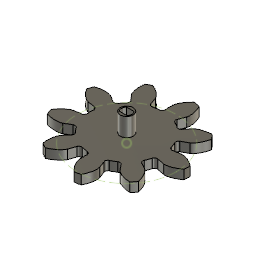
Master Gear (Autodesk Fusion 360 design; units mm, degrees)
description: Spur Gear; Module: 6.000000; Num Teeth: 9; Pressure Angle: 20.000000; Backlash: 0.00 mm
Autodesk Fusion 360 part; units mm, degrees
(part 1 of 2)
sketch "Sketch1" plane through (0, 0, 0) normal (0, 0, 1) x (1, 0, 0) in component "Spur Gear (9 teeth)"
  circle A0 centre (0, 0) radius 19.7492
extrude "Extrude1" add sketch "Sketch1" along normal blind 5 in component "Spur Gear (9 teeth)"
sketch "Sketch2" plane through (0, 0, 0) normal (0, 0, 1) x (1, 0, 0) in component "Spur Gear (9 teeth)"
  spline S0 degree 5 poles (24.9178, -4.7777) (24.9406, -4.782) (24.9862, -4.7899) (25.0549, -4.7992) (25.1471, -4.8069) (25.263, -4.8101) (25.3794, -4.8088) (25.4962, -4.8047) (25.6131, -4.7991) (25.7301, -4.7925) (25.8472, -4.7846) (25.9644, -4.7752) (26.0817, -4.7637) (26.1992, -4.7499) (26.3168, -4.7338) (26.4345, -4.7156) (26.5523, -4.6956) (26.67, -4.6741) (26.7878, -4.6513) (26.9056, -4.6272) (27.0233, -4.6018) (27.1411, -4.5751) (27.2588, -4.5468) (27.3765, -4.5171) (27.4941, -4.486) (27.6117, -4.4534) (27.7292, -4.4196) (27.8467, -4.3845) (27.9641, -4.3482) (28.0813, -4.3107) (28.1985, -4.272) (28.3156, -4.2321) (28.4326, -4.191) (28.5495, -4.1487) (28.6662, -4.1053) (28.7828, -4.0606) (28.8993, -4.0149) (29.0157, -3.968) (29.1319, -3.9201) (29.2479, -3.8711) (29.3638, -3.821) (29.4795, -3.7698) (29.595, -3.7175) (29.7104, -3.6643) (29.8256, -3.6099) (29.9406, -3.5546) (30.0554, -3.4982) (30.17, -3.4408) (30.2844, -3.3824) (30.3986, -3.323) (30.5125, -3.2626) (30.6263, -3.2013) (30.7398, -3.139) (30.8531, -3.0757) (30.9662, -3.0114) (31.079, -2.9462) (31.1916, -2.8801) (31.3039, -2.8131) (31.416, -2.7451) (31.5279, -2.6762) (31.6394, -2.6063) (31.7507, -2.5356) (31.8618, -2.464) (31.9725, -2.3914) (32.083, -2.318) (32.1932, -2.2437) (32.3031, -2.1685) (32.4127, -2.0925) (32.522, -2.0156) (32.6311, -1.9378) (32.7398, -1.8592) (32.8265, -1.7956) (32.8914, -1.7475) (32.9346, -1.7153) (32.9562, -1.6991) knots 0 0 0 0 0 0 0.01428571 0.02857143 0.04285714 0.05714286 0.07142857 0.08571429 0.1 0.11428571 0.12857143 0.14285714 0.15714286 0.17142857 0.18571429 0.2 0.21428571 0.22857143 0.24285714 0.25714286 0.27142857 0.28571429 0.3 0.31428571 0.32857143 0.34285714 0.35714286 0.37142857 0.38571429 0.4 0.41428571 0.42857143 0.44285714 0.45714286 0.47142857 0.48571429 0.5 0.51428571 0.52857143 0.54285714 0.55714286 0.57142857 0.58571429 0.6 0.61428571 0.62857143 0.64285714 0.65714286 0.67142857 0.68571429 0.7 0.71428571 0.72857143 0.74285714 0.75714286 0.77142857 0.78571429 0.8 0.81428571 0.82857143 0.84285714 0.85714286 0.87142857 0.88571429 0.9 0.91428571 0.92857143 0.94285714 0.95714286 0.97142857 0.98571429 1 1 1 1 1 1
  spline S1 degree 5 poles (24.9178, 4.7777) (24.9406, 4.782) (24.9862, 4.7899) (25.0549, 4.7992) (25.1471, 4.8069) (25.263, 4.8101) (25.3794, 4.8088) (25.4962, 4.8047) (25.6131, 4.7991) (25.7301, 4.7925) (25.8472, 4.7846) (25.9644, 4.7752) (26.0817, 4.7637) (26.1992, 4.7499) (26.3168, 4.7338) (26.4345, 4.7156) (26.5523, 4.6956) (26.67, 4.6741) (26.7878, 4.6513) (26.9056, 4.6272) (27.0233, 4.6018) (27.1411, 4.5751) (27.2588, 4.5468) (27.3765, 4.5171) (27.4941, 4.486) (27.6117, 4.4534) (27.7292, 4.4196) (27.8467, 4.3845) (27.9641, 4.3482) (28.0813, 4.3107) (28.1985, 4.272) (28.3156, 4.2321) (28.4326, 4.191) (28.5495, 4.1487) (28.6662, 4.1053) (28.7828, 4.0606) (28.8993, 4.0149) (29.0157, 3.968) (29.1319, 3.9201) (29.2479, 3.8711) (29.3638, 3.821) (29.4795, 3.7698) (29.595, 3.7175) (29.7104, 3.6643) (29.8256, 3.6099) (29.9406, 3.5546) (30.0554, 3.4982) (30.17, 3.4408) (30.2844, 3.3824) (30.3986, 3.323) (30.5125, 3.2626) (30.6263, 3.2013) (30.7398, 3.139) (30.8531, 3.0757) (30.9662, 3.0114) (31.079, 2.9462) (31.1916, 2.8801) (31.3039, 2.8131) (31.416, 2.7451) (31.5279, 2.6762) (31.6394, 2.6063) (31.7507, 2.5356) (31.8618, 2.464) (31.9725, 2.3914) (32.083, 2.318) (32.1932, 2.2437) (32.3031, 2.1685) (32.4127, 2.0925) (32.522, 2.0156) (32.6311, 1.9378) (32.7398, 1.8592) (32.8265, 1.7956) (32.8914, 1.7475) (32.9346, 1.7153) (32.9562, 1.6991) knots 0 0 0 0 0 0 0.01428571 0.02857143 0.04285714 0.05714286 0.07142857 0.08571429 0.1 0.11428571 0.12857143 0.14285714 0.15714286 0.17142857 0.18571429 0.2 0.21428571 0.22857143 0.24285714 0.25714286 0.27142857 0.28571429 0.3 0.31428571 0.32857143 0.34285714 0.35714286 0.37142857 0.38571429 0.4 0.41428571 0.42857143 0.44285714 0.45714286 0.47142857 0.48571429 0.5 0.51428571 0.52857143 0.54285714 0.55714286 0.57142857 0.58571429 0.6 0.61428571 0.62857143 0.64285714 0.65714286 0.67142857 0.68571429 0.7 0.71428571 0.72857143 0.74285714 0.75714286 0.77142857 0.78571429 0.8 0.81428571 0.82857143 0.84285714 0.85714286 0.87142857 0.88571429 0.9 0.91428571 0.92857143 0.94285714 0.95714286 0.97142857 0.98571429 1 1 1 1 1 1
  arc A0 (32.9562, -1.6991) -> (32.9562, 1.6991) centre (0, 0) ccw
  line L0 (19.3861, -3.7189) -> (24.9178, -4.7777)
  line L1 (19.3861, 3.7189) -> (24.9178, 4.7777)
  line L2 (19.3861, -3.7189) -> (19.3861, 3.7189)
  point P0 (25.4672, -4.8054)
  point P1 (26.0282, -4.7687)
  point P2 (26.5965, -4.6873)
  point P3 (27.1699, -4.5679)
  point P4 (27.7472, -4.414)
  point P5 (28.3272, -4.2278)
  point P6 (28.909, -4.0108)
  point P7 (29.4915, -3.7641)
  point P8 (30.0739, -3.4887)
  point P9 (30.6555, -3.1851)
  point P10 (31.2353, -2.8539)
  point P11 (31.8125, -2.4956)
  point P12 (32.3864, -2.1106)
  point P13 (25.4672, 4.8054)
  point P14 (26.0282, 4.7687)
  point P15 (26.5965, 4.6873)
  point P16 (27.1699, 4.5679)
  point P17 (27.7472, 4.414)
  point P18 (28.3272, 4.2278)
  point P19 (28.909, 4.0108)
  point P20 (29.4915, 3.7641)
  point P21 (30.0739, 3.4887)
  point P22 (30.6555, 3.1851)
  point P23 (31.2353, 2.8539)
  point P24 (31.8125, 2.4956)
  point P25 (32.3864, 2.1106)
extrude "Extrude2" add sketch "Sketch2" along normal blind 5 in component "Spur Gear (9 teeth)"
fillet "Fillet1" radius 1.5875 2 edges at (19.3955, -3.7207, 2.5) (19.3955, 3.7207, 2.5) in component "Spur Gear (9 teeth)"
pattern_circular "C-Pattern1" count 9 over 360 about axis through (0, 0, 0) along (0, 0, 1) of "Extrude2", "Fillet1" in component "Spur Gear (9 teeth)"
sketch "Sketch3" plane through (0, 0, 0) normal (0, 0, 1) x (1, 0, 0) in component "Spur Gear (9 teeth)"
  circle A0 centre (0, 0) radius 27 construction
sketch "Sketch1 (2)" plane through (0, 0, 5) normal (0, 0, 1) x (-1, 0, 0)
  arc A0 (-17.9169, 8.3075) -> (-19.0651, 5.1529) centre (0, 0) ccw
  arc A1 (-20.896, 4.0079) -> (-19.0651, 5.1529) centre (-20.5976, 5.5671) ccw
  line L0 (-20.896, 4.0079) -> (-24.9178, 4.7777)
  spline S0 degree 5 poles (-24.9178, 4.7777) (-24.9406, 4.782) (-24.9862, 4.7899) (-25.0549, 4.7992) (-25.1471, 4.8069) (-25.263, 4.8101) (-25.3794, 4.8088) (-25.4962, 4.8047) (-25.6131, 4.7991) (-25.7301, 4.7925) (-25.8472, 4.7846) (-25.9644, 4.7752) (-26.0817, 4.7637) (-26.1992, 4.7499) (-26.3168, 4.7338) (-26.4345, 4.7156) (-26.5523, 4.6956) (-26.67, 4.6741) (-26.7878, 4.6513) (-26.9056, 4.6272) (-27.0233, 4.6018) (-27.1411, 4.5751) (-27.2588, 4.5468) (-27.3765, 4.5171) (-27.4941, 4.486) (-27.6117, 4.4534) (-27.7292, 4.4196) (-27.8467, 4.3845) (-27.9641, 4.3482) (-28.0813, 4.3107) (-28.1985, 4.272) (-28.3156, 4.2321) (-28.4326, 4.191) (-28.5495, 4.1487) (-28.6662, 4.1053) (-28.7828, 4.0606) (-28.8993, 4.0149) (-29.0157, 3.968) (-29.1319, 3.9201) (-29.2479, 3.8711) (-29.3638, 3.821) (-29.4795, 3.7698) (-29.595, 3.7175) (-29.7104, 3.6643) (-29.8256, 3.6099) (-29.9406, 3.5546) (-30.0554, 3.4982) (-30.17, 3.4408) (-30.2844, 3.3824) (-30.3986, 3.323) (-30.5125, 3.2626) (-30.6263, 3.2013) (-30.7398, 3.139) (-30.8531, 3.0757) (-30.9662, 3.0114) (-31.079, 2.9462) (-31.1916, 2.8801) (-31.3039, 2.8131) (-31.416, 2.7451) (-31.5279, 2.6762) (-31.6394, 2.6063) (-31.7507, 2.5356) (-31.8618, 2.464) (-31.9725, 2.3914) (-32.083, 2.318) (-32.1932, 2.2437) (-32.3031, 2.1685) (-32.4127, 2.0925) (-32.522, 2.0156) (-32.6311, 1.9378) (-32.7398, 1.8592) (-32.8265, 1.7956) (-32.8914, 1.7475) (-32.9346, 1.7153) (-32.9562, 1.6991) knots 0 0 0 0 0 0 0.01428571 0.02857143 0.04285714 0.05714286 0.07142857 0.08571429 0.1 0.11428571 0.12857143 0.14285714 0.15714286 0.17142857 0.18571429 0.2 0.21428571 0.22857143 0.24285714 0.25714286 0.27142857 0.28571429 0.3 0.31428571 0.32857143 0.34285714 0.35714286 0.37142857 0.38571429 0.4 0.41428571 0.42857143 0.44285714 0.45714286 0.47142857 0.48571429 0.5 0.51428571 0.52857143 0.54285714 0.55714286 0.57142857 0.58571429 0.6 0.61428571 0.62857143 0.64285714 0.65714286 0.67142857 0.68571429 0.7 0.71428571 0.72857143 0.74285714 0.75714286 0.77142857 0.78571429 0.8 0.81428571 0.82857143 0.84285714 0.85714286 0.87142857 0.88571429 0.9 0.91428571 0.92857143 0.94285714 0.95714286 0.97142857 0.98571429 1 1 1 1 1 1
  arc A2 (-32.9562, 1.6991) -> (-32.9562, -1.6991) centre (0, 0) ccw
  spline S1 degree 5 poles (-32.9562, -1.6991) (-32.9346, -1.7153) (-32.8914, -1.7475) (-32.8265, -1.7956) (-32.7398, -1.8592) (-32.6311, -1.9378) (-32.522, -2.0156) (-32.4127, -2.0925) (-32.3031, -2.1685) (-32.1932, -2.2437) (-32.083, -2.318) (-31.9725, -2.3914) (-31.8618, -2.464) (-31.7507, -2.5356) (-31.6394, -2.6063) (-31.5279, -2.6762) (-31.416, -2.7451) (-31.3039, -2.8131) (-31.1916, -2.8801) (-31.079, -2.9462) (-30.9662, -3.0114) (-30.8531, -3.0757) (-30.7398, -3.139) (-30.6263, -3.2013) (-30.5125, -3.2626) (-30.3986, -3.323) (-30.2844, -3.3824) (-30.17, -3.4408) (-30.0554, -3.4982) (-29.9406, -3.5546) (-29.8256, -3.6099) (-29.7104, -3.6643) (-29.595, -3.7175) (-29.4795, -3.7698) (-29.3638, -3.821) (-29.2479, -3.8711) (-29.1319, -3.9201) (-29.0157, -3.968) (-28.8993, -4.0149) (-28.7828, -4.0606) (-28.6662, -4.1053) (-28.5495, -4.1487) (-28.4326, -4.191) (-28.3156, -4.2321) (-28.1985, -4.272) (-28.0813, -4.3107) (-27.9641, -4.3482) (-27.8467, -4.3845) (-27.7292, -4.4196) (-27.6117, -4.4534) (-27.4941, -4.486) (-27.3765, -4.5171) (-27.2588, -4.5468) (-27.1411, -4.5751) (-27.0233, -4.6018) (-26.9056, -4.6272) (-26.7878, -4.6513) (-26.67, -4.6741) (-26.5523, -4.6956) (-26.4345, -4.7156) (-26.3168, -4.7338) (-26.1992, -4.7499) (-26.0817, -4.7637) (-25.9644, -4.7752) (-25.8472, -4.7846) (-25.7301, -4.7925) (-25.6131, -4.7991) (-25.4962, -4.8047) (-25.3794, -4.8088) (-25.263, -4.8101) (-25.1471, -4.8069) (-25.0549, -4.7992) (-24.9862, -4.7899) (-24.9406, -4.782) (-24.9178, -4.7777) knots -1 -1 -1 -1 -1 -1 -0.98571429 -0.97142857 -0.95714286 -0.94285714 -0.92857143 -0.91428571 -0.9 -0.88571429 -0.87142857 -0.85714286 -0.84285714 -0.82857143 -0.81428571 -0.8 -0.78571429 -0.77142857 -0.75714286 -0.74285714 -0.72857143 -0.71428571 -0.7 -0.68571429 -0.67142857 -0.65714286 -0.64285714 -0.62857143 -0.61428571 -0.6 -0.58571429 -0.57142857 -0.55714286 -0.54285714 -0.52857143 -0.51428571 -0.5 -0.48571429 -0.47142857 -0.45714286 -0.44285714 -0.42857143 -0.41428571 -0.4 -0.38571429 -0.37142857 -0.35714286 -0.34285714 -0.32857143 -0.31428571 -0.3 -0.28571429 -0.27142857 -0.25714286 -0.24285714 -0.22857143 -0.21428571 -0.2 -0.18571429 -0.17142857 -0.15714286 -0.14285714 -0.12857143 -0.11428571 -0.1 -0.08571429 -0.07142857 -0.05714286 -0.04285714 -0.02857143 -0.01428571 0 0 0 0 0 0
  line L1 (-24.9178, -4.7777) -> (-20.896, -4.0079)
  arc A3 (-19.0651, -5.1529) -> (-20.896, -4.0079) centre (-20.5976, -5.5671) ccw
  arc A4 (-19.0651, -5.1529) -> (-17.9169, -8.3075) centre (0, 0) ccw
  arc A5 (-18.5835, -10.3615) -> (-17.9169, -8.3075) centre (-19.3572, -8.9753) ccw
  line L2 (-18.5835, -10.3615) -> (-22.1592, -12.357)
  spline S2 degree 5 poles (-22.1592, -12.357) (-22.1794, -12.3683) (-22.2194, -12.3916) (-22.2781, -12.4286) (-22.3536, -12.4819) (-22.4445, -12.554) (-22.5328, -12.6298) (-22.6196, -12.708) (-22.7055, -12.7874) (-22.7909, -12.8677) (-22.8756, -12.949) (-22.9593, -13.0316) (-23.0418, -13.1158) (-23.1229, -13.2019) (-23.2027, -13.2899) (-23.2811, -13.3795) (-23.3585, -13.4705) (-23.4349, -13.5626) (-23.5105, -13.6558) (-23.5852, -13.7499) (-23.6591, -13.845) (-23.7321, -13.9412) (-23.8041, -14.0385) (-23.8751, -14.1369) (-23.9452, -14.2364) (-24.0144, -14.3369) (-24.0827, -14.4384) (-24.1501, -14.5408) (-24.2167, -14.644) (-24.2824, -14.7482) (-24.3473, -14.8531) (-24.4114, -14.959) (-24.4746, -15.0656) (-24.5369, -15.1732) (-24.5984, -15.2815) (-24.6591, -15.3906) (-24.7189, -15.5005) (-24.7779, -15.6112) (-24.8361, -15.7226) (-24.8935, -15.8348) (-24.95, -15.9476) (-25.0058, -16.0612) (-25.0607, -16.1755) (-25.1148, -16.2905) (-25.1681, -16.4061) (-25.2206, -16.5225) (-25.2723, -16.6395) (-25.3232, -16.7571) (-25.3733, -16.8754) (-25.4226, -16.9942) (-25.4711, -17.1138) (-25.5188, -17.2339) (-25.5658, -17.3546) (-25.6119, -17.4759) (-25.6572, -17.5978) (-25.7017, -17.7203) (-25.7455, -17.8433) (-25.7884, -17.9669) (-25.8306, -18.091) (-25.8719, -18.2157) (-25.9125, -18.3409) (-25.9523, -18.4666) (-25.9913, -18.5928) (-26.0296, -18.7196) (-26.067, -18.8469) (-26.1037, -18.9746) (-26.1395, -19.1029) (-26.1746, -19.2316) (-26.2089, -19.3607) (-26.2424, -19.4904) (-26.2752, -19.6205) (-26.3007, -19.725) (-26.3196, -19.8035) (-26.332, -19.856) (-26.3381, -19.8822) knots 0 0 0 0 0 0 0.01428571 0.02857143 0.04285714 0.05714286 0.07142857 0.08571429 0.1 0.11428571 0.12857143 0.14285714 0.15714286 0.17142857 0.18571429 0.2 0.21428571 0.22857143 0.24285714 0.25714286 0.27142857 0.28571429 0.3 0.31428571 0.32857143 0.34285714 0.35714286 0.37142857 0.38571429 0.4 0.41428571 0.42857143 0.44285714 0.45714286 0.47142857 0.48571429 0.5 0.51428571 0.52857143 0.54285714 0.55714286 0.57142857 0.58571429 0.6 0.61428571 0.62857143 0.64285714 0.65714286 0.67142857 0.68571429 0.7 0.71428571 0.72857143 0.74285714 0.75714286 0.77142857 0.78571429 0.8 0.81428571 0.82857143 0.84285714 0.85714286 0.87142857 0.88571429 0.9 0.91428571 0.92857143 0.94285714 0.95714286 0.97142857 0.98571429 1 1 1 1 1 1
  arc A6 (-26.3381, -19.8822) -> (-24.1537, -22.4855) centre (0, 0) ccw
  spline S3 degree 5 poles (-24.1537, -22.4855) (-24.1268, -22.484) (-24.073, -22.4809) (-23.9924, -22.476) (-23.8851, -22.4689) (-23.7512, -22.4593) (-23.6177, -22.4488) (-23.4846, -22.4374) (-23.3517, -22.4252) (-23.2192, -22.4122) (-23.087, -22.3983) (-22.9552, -22.3835) (-22.8237, -22.3679) (-22.6926, -22.3514) (-22.5619, -22.334) (-22.4315, -22.3158) (-22.3016, -22.2967) (-22.172, -22.2767) (-22.0429, -22.2559) (-21.9141, -22.2342) (-21.7858, -22.2116) (-21.6579, -22.1881) (-21.5304, -22.1638) (-21.4034, -22.1385) (-21.2768, -22.1124) (-21.1507, -22.0854) (-21.025, -22.0575) (-20.8998, -22.0287) (-20.7752, -21.999) (-20.651, -21.9684) (-20.5273, -21.9369) (-20.4041, -21.9045) (-20.2815, -21.8711) (-20.1594, -21.8369) (-20.0379, -21.8017) (-19.9169, -21.7656) (-19.7965, -21.7286) (-19.6767, -21.6906) (-19.5574, -21.6517) (-19.4388, -21.6119) (-19.3208, -21.5711) (-19.2034, -21.5293) (-19.0867, -21.4866) (-18.9707, -21.4429) (-18.8553, -21.3982) (-18.7407, -21.3525) (-18.6267, -21.3059) (-18.5135, -21.2582) (-18.401, -21.2096) (-18.2892, -21.16) (-18.1782, -21.1093) (-18.068, -21.0576) (-17.9588, -21.0047) (-17.8505, -20.9506) (-17.7431, -20.8955) (-17.6365, -20.8392) (-17.5309, -20.782) (-17.426, -20.7237) (-17.322, -20.6645) (-17.2189, -20.6041) (-17.1171, -20.5424) (-17.0166, -20.4792) (-16.9177, -20.4142) (-16.8204, -20.3476) (-16.7246, -20.2795) (-16.6299, -20.2102) (-16.5359, -20.1401) (-16.4428, -20.0692) (-16.3507, -19.9973) (-16.2607, -19.9235) (-16.174, -19.8466) (-16.1083, -19.7814) (-16.0617, -19.7301) (-16.0318, -19.6947) (-16.0171, -19.6768) knots -1 -1 -1 -1 -1 -1 -0.98571429 -0.97142857 -0.95714286 -0.94285714 -0.92857143 -0.91428571 -0.9 -0.88571429 -0.87142857 -0.85714286 -0.84285714 -0.82857143 -0.81428571 -0.8 -0.78571429 -0.77142857 -0.75714286 -0.74285714 -0.72857143 -0.71428571 -0.7 -0.68571429 -0.67142857 -0.65714286 -0.64285714 -0.62857143 -0.61428571 -0.6 -0.58571429 -0.57142857 -0.55714286 -0.54285714 -0.52857143 -0.51428571 -0.5 -0.48571429 -0.47142857 -0.45714286 -0.44285714 -0.42857143 -0.41428571 -0.4 -0.38571429 -0.37142857 -0.35714286 -0.34285714 -0.32857143 -0.31428571 -0.3 -0.28571429 -0.27142857 -0.25714286 -0.24285714 -0.22857143 -0.21428571 -0.2 -0.18571429 -0.17142857 -0.15714286 -0.14285714 -0.12857143 -0.11428571 -0.1 -0.08571429 -0.07142857 -0.05714286 -0.04285714 -0.02857143 -0.01428571 0 0 0 0 0 0
  line L3 (-16.0171, -19.6768) -> (-13.4311, -16.502)
  arc A7 (-11.2925, -16.2022) -> (-13.4311, -16.502) centre (-12.2002, -17.5045) ccw
  arc A8 (-11.2925, -16.2022) -> (-8.3852, -17.8807) centre (0, 0) ccw
  arc A9 (-7.5756, -19.8826) -> (-8.3852, -17.8807) centre (-9.0593, -19.318) ccw
  line L4 (-7.5756, -19.8826) -> (-9.032, -23.7096)
  spline S4 degree 5 poles (-9.032, -23.7096) (-9.0402, -23.7313) (-9.0559, -23.7749) (-9.0771, -23.8409) (-9.1006, -23.9303) (-9.1239, -24.0439) (-9.1428, -24.1588) (-9.159, -24.2745) (-9.1738, -24.3906) (-9.1876, -24.507) (-9.2003, -24.6237) (-9.2113, -24.7407) (-9.2204, -24.8583) (-9.2272, -24.9764) (-9.2317, -25.095) (-9.2342, -25.2141) (-9.235, -25.3335) (-9.2343, -25.4532) (-9.2323, -25.5732) (-9.229, -25.6933) (-9.2245, -25.8137) (-9.2186, -25.9343) (-9.2112, -26.0551) (-9.2024, -26.1762) (-9.1921, -26.2974) (-9.1805, -26.4189) (-9.1676, -26.5405) (-9.1534, -26.6623) (-9.138, -26.7842) (-9.1215, -26.9062) (-9.1037, -27.0283) (-9.0848, -27.1506) (-9.0646, -27.2729) (-9.0432, -27.3953) (-9.0207, -27.5178) (-8.997, -27.6404) (-8.9722, -27.7631) (-8.9463, -27.8858) (-8.9192, -28.0086) (-8.8911, -28.1313) (-8.8619, -28.2542) (-8.8316, -28.377) (-8.8002, -28.4999) (-8.7677, -28.6227) (-8.7342, -28.7456) (-8.6997, -28.8685) (-8.6641, -28.9913) (-8.6275, -29.1141) (-8.5898, -29.2369) (-8.5512, -29.3597) (-8.5115, -29.4824) (-8.4708, -29.6051) (-8.4292, -29.7277) (-8.3865, -29.8503) (-8.3429, -29.9728) (-8.2983, -30.0953) (-8.2527, -30.2176) (-8.2062, -30.3399) (-8.1587, -30.4621) (-8.1103, -30.5842) (-8.0609, -30.7062) (-8.0105, -30.8281) (-7.9593, -30.9499) (-7.9071, -31.0715) (-7.854, -31.1931) (-7.7999, -31.3145) (-7.745, -31.4358) (-7.6891, -31.557) (-7.6323, -31.678) (-7.5747, -31.7988) (-7.5161, -31.9195) (-7.4686, -32.016) (-7.4325, -32.0883) (-7.4083, -32.1364) (-7.3961, -32.1605) knots 0 0 0 0 0 0 0.01428571 0.02857143 0.04285714 0.05714286 0.07142857 0.08571429 0.1 0.11428571 0.12857143 0.14285714 0.15714286 0.17142857 0.18571429 0.2 0.21428571 0.22857143 0.24285714 0.25714286 0.27142857 0.28571429 0.3 0.31428571 0.32857143 0.34285714 0.35714286 0.37142857 0.38571429 0.4 0.41428571 0.42857143 0.44285714 0.45714286 0.47142857 0.48571429 0.5 0.51428571 0.52857143 0.54285714 0.55714286 0.57142857 0.58571429 0.6 0.61428571 0.62857143 0.64285714 0.65714286 0.67142857 0.68571429 0.7 0.71428571 0.72857143 0.74285714 0.75714286 0.77142857 0.78571429 0.8 0.81428571 0.82857143 0.84285714 0.85714286 0.87142857 0.88571429 0.9 0.91428571 0.92857143 0.94285714 0.95714286 0.97142857 0.98571429 1 1 1 1 1 1
  arc A10 (-7.3961, -32.1605) -> (-4.0495, -32.7506) centre (0, 0) ccw
  spline S5 degree 5 poles (-4.0495, -32.7506) (-4.0298, -32.7321) (-3.9906, -32.6952) (-3.932, -32.6396) (-3.8543, -32.5652) (-3.758, -32.4718) (-3.6624, -32.378) (-3.5677, -32.2837) (-3.4738, -32.1889) (-3.3807, -32.0937) (-3.2884, -31.9981) (-3.1969, -31.9021) (-3.1062, -31.8056) (-3.0164, -31.7087) (-2.9274, -31.6113) (-2.8393, -31.5136) (-2.752, -31.4154) (-2.6656, -31.3169) (-2.58, -31.2179) (-2.4953, -31.1185) (-2.4115, -31.0187) (-2.3286, -30.9185) (-2.2466, -30.8179) (-2.1656, -30.7169) (-2.0854, -30.6155) (-2.0061, -30.5138) (-1.9278, -30.4116) (-1.8504, -30.3091) (-1.774, -30.2062) (-1.6986, -30.1029) (-1.6241, -29.9993) (-1.5506, -29.8953) (-1.4781, -29.791) (-1.4065, -29.6862) (-1.3361, -29.5812) (-1.2666, -29.4758) (-1.1981, -29.37) (-1.1308, -29.2639) (-1.0644, -29.1575) (-0.9991, -29.0507) (-0.935, -28.9436) (-0.8719, -28.8362) (-0.8099, -28.7284) (-0.7492, -28.6203) (-0.6895, -28.512) (-0.6311, -28.4033) (-0.5738, -28.2943) (-0.5176, -28.185) (-0.4627, -28.0754) (-0.4089, -27.9655) (-0.3565, -27.8554) (-0.3054, -27.7449) (-0.2557, -27.6342) (-0.2074, -27.5232) (-0.1606, -27.4119) (-0.1152, -27.3003) (-0.071, -27.1885) (-0.0281, -27.0765) (0.0135, -26.9643) (0.0536, -26.8518) (0.092, -26.739) (0.1283, -26.626) (0.1623, -26.5127) (0.194, -26.3991) (0.2236, -26.2853) (0.2517, -26.1714) (0.2785, -26.0573) (0.3043, -25.9431) (0.3286, -25.8289) (0.3502, -25.7145) (0.3671, -25.5998) (0.3756, -25.5077) (0.3783, -25.4384) (0.3785, -25.3921) (0.3781, -25.3689) knots -1 -1 -1 -1 -1 -1 -0.98571429 -0.97142857 -0.95714286 -0.94285714 -0.92857143 -0.91428571 -0.9 -0.88571429 -0.87142857 -0.85714286 -0.84285714 -0.82857143 -0.81428571 -0.8 -0.78571429 -0.77142857 -0.75714286 -0.74285714 -0.72857143 -0.71428571 -0.7 -0.68571429 -0.67142857 -0.65714286 -0.64285714 -0.62857143 -0.61428571 -0.6 -0.58571429 -0.57142857 -0.55714286 -0.54285714 -0.52857143 -0.51428571 -0.5 -0.48571429 -0.47142857 -0.45714286 -0.44285714 -0.42857143 -0.41428571 -0.4 -0.38571429 -0.37142857 -0.35714286 -0.34285714 -0.32857143 -0.31428571 -0.3 -0.28571429 -0.27142857 -0.25714286 -0.24285714 -0.22857143 -0.21428571 -0.2 -0.18571429 -0.17142857 -0.15714286 -0.14285714 -0.12857143 -0.11428571 -0.1 -0.08571429 -0.07142857 -0.05714286 -0.04285714 -0.02857143 -0.01428571 0 0 0 0 0 0
  line L5 (0.3781, -25.3689) -> (0.3185, -21.2746)
  arc A11 (1.764, -19.6703) -> (0.3185, -21.2746) centre (1.9058, -21.2514) ccw
  arc A12 (1.764, -19.6703) -> (5.07, -19.0873) centre (0, 0) ccw
  arc A13 (6.9771, -20.1005) -> (5.07, -19.0873) centre (5.4776, -20.6216) ccw
  line L6 (6.9771, -20.1005) -> (8.3213, -23.9683)
  spline S6 degree 5 poles (8.3213, -23.9683) (8.3289, -23.9902) (8.3449, -24.0336) (8.3712, -24.0978) (8.4106, -24.1815) (8.4658, -24.2835) (8.5252, -24.3836) (8.5871, -24.4827) (8.6504, -24.5811) (8.7147, -24.6791) (8.78, -24.7766) (8.8467, -24.8734) (8.9154, -24.9693) (8.9861, -25.0641) (9.0589, -25.1579) (9.1335, -25.2507) (9.2097, -25.3427) (9.2871, -25.434) (9.3658, -25.5246) (9.4455, -25.6145) (9.5264, -25.7038) (9.6084, -25.7924) (9.6917, -25.8802) (9.7763, -25.9673) (9.8621, -26.0536) (9.949, -26.1391) (10.0371, -26.224) (10.1262, -26.3082) (10.2164, -26.3917) (10.3075, -26.4745) (10.3996, -26.5566) (10.4927, -26.6381) (10.5868, -26.7189) (10.6818, -26.7989) (10.7779, -26.8783) (10.8748, -26.957) (10.9727, -27.035) (11.0714, -27.1123) (11.171, -27.189) (11.2715, -27.265) (11.3728, -27.3403) (11.475, -27.4149) (11.578, -27.4888) (11.6819, -27.5621) (11.7865, -27.6347) (11.8919, -27.7066) (11.9982, -27.7778) (12.1052, -27.8484) (12.2129, -27.9182) (12.3215, -27.9874) (12.4307, -28.0559) (12.5408, -28.1238) (12.6515, -28.1909) (12.763, -28.2574) (12.8751, -28.3232) (12.988, -28.3883) (13.1016, -28.4528) (13.2158, -28.5165) (13.3307, -28.5796) (13.4463, -28.642) (13.5626, -28.7037) (13.6795, -28.7647) (13.797, -28.8251) (13.9152, -28.8847) (14.034, -28.9437) (14.1535, -29.002) (14.2736, -29.0596) (14.3942, -29.1165) (14.5155, -29.1727) (14.6373, -29.2282) (14.7598, -29.2831) (14.8582, -29.3264) (14.9323, -29.3586) (14.9818, -29.3799) (15.0066, -29.3905) knots 0 0 0 0 0 0 0.01428571 0.02857143 0.04285714 0.05714286 0.07142857 0.08571429 0.1 0.11428571 0.12857143 0.14285714 0.15714286 0.17142857 0.18571429 0.2 0.21428571 0.22857143 0.24285714 0.25714286 0.27142857 0.28571429 0.3 0.31428571 0.32857143 0.34285714 0.35714286 0.37142857 0.38571429 0.4 0.41428571 0.42857143 0.44285714 0.45714286 0.47142857 0.48571429 0.5 0.51428571 0.52857143 0.54285714 0.55714286 0.57142857 0.58571429 0.6 0.61428571 0.62857143 0.64285714 0.65714286 0.67142857 0.68571429 0.7 0.71428571 0.72857143 0.74285714 0.75714286 0.77142857 0.78571429 0.8 0.81428571 0.82857143 0.84285714 0.85714286 0.87142857 0.88571429 0.9 0.91428571 0.92857143 0.94285714 0.95714286 0.97142857 0.98571429 1 1 1 1 1 1
  arc A14 (15.0066, -29.3905) -> (17.9496, -27.6914) centre (0, 0) ccw
  spline S7 degree 5 poles (17.9496, -27.6914) (17.9528, -27.6646) (17.9591, -27.611) (17.9683, -27.5308) (17.98, -27.4239) (17.9937, -27.2904) (18.0066, -27.1571) (18.0185, -27.024) (18.0296, -26.8911) (18.0397, -26.7583) (18.049, -26.6257) (18.0573, -26.4933) (18.0647, -26.3611) (18.0713, -26.2291) (18.0769, -26.0974) (18.0816, -25.9659) (18.0853, -25.8346) (18.0882, -25.7035) (18.0901, -25.5727) (18.091, -25.4421) (18.0911, -25.3118) (18.0902, -25.1818) (18.0883, -25.052) (18.0855, -24.9225) (18.0818, -24.7933) (18.0771, -24.6644) (18.0714, -24.5358) (18.0648, -24.4076) (18.0572, -24.2796) (18.0486, -24.152) (18.0391, -24.0247) (18.0285, -23.8978) (18.017, -23.7713) (18.0045, -23.6451) (17.9909, -23.5193) (17.9764, -23.3939) (17.9608, -23.2689) (17.9443, -23.1443) (17.9267, -23.0201) (17.908, -22.8963) (17.8884, -22.773) (17.8676, -22.6502) (17.8458, -22.5279) (17.8229, -22.406) (17.7989, -22.2847) (17.7738, -22.1638) (17.7477, -22.0435) (17.7204, -21.9237) (17.6921, -21.8044) (17.6626, -21.6857) (17.632, -21.5676) (17.6002, -21.4501) (17.5671, -21.3334) (17.5327, -21.2173) (17.497, -21.102) (17.4601, -20.9873) (17.4221, -20.8733) (17.3829, -20.7599) (17.3426, -20.6472) (17.3011, -20.5352) (17.258, -20.4242) (17.2131, -20.3142) (17.1664, -20.2056) (17.1177, -20.0982) (17.0672, -19.992) (17.0154, -19.8867) (16.9627, -19.782) (16.909, -19.678) (16.8542, -19.5748) (16.7972, -19.4733) (16.7365, -19.3746) (16.6837, -19.2986) (16.6413, -19.2438) (16.6116, -19.2082) (16.5965, -19.1906) knots -1 -1 -1 -1 -1 -1 -0.98571429 -0.97142857 -0.95714286 -0.94285714 -0.92857143 -0.91428571 -0.9 -0.88571429 -0.87142857 -0.85714286 -0.84285714 -0.82857143 -0.81428571 -0.8 -0.78571429 -0.77142857 -0.75714286 -0.74285714 -0.72857143 -0.71428571 -0.7 -0.68571429 -0.67142857 -0.65714286 -0.64285714 -0.62857143 -0.61428571 -0.6 -0.58571429 -0.57142857 -0.55714286 -0.54285714 -0.52857143 -0.51428571 -0.5 -0.48571429 -0.47142857 -0.45714286 -0.44285714 -0.42857143 -0.41428571 -0.4 -0.38571429 -0.37142857 -0.35714286 -0.34285714 -0.32857143 -0.31428571 -0.3 -0.28571429 -0.27142857 -0.25714286 -0.24285714 -0.22857143 -0.21428571 -0.2 -0.18571429 -0.17142857 -0.15714286 -0.14285714 -0.12857143 -0.11428571 -0.1 -0.08571429 -0.07142857 -0.05714286 -0.04285714 -0.02857143 -0.01428571 0 0 0 0 0 0
  line L7 (16.5965, -19.1906) -> (13.919, -16.0926)
  arc A15 (13.9951, -13.9344) -> (13.919, -16.0926) centre (15.1201, -15.0545) ccw
  arc A16 (13.9951, -13.9344) -> (16.153, -11.3628) centre (0, 0) ccw
  arc A17 (18.2651, -10.9131) -> (16.153, -11.3628) centre (17.4514, -12.2762) ccw
  line L8 (18.2651, -10.9131) -> (21.781, -13.0119)
  spline S8 degree 5 poles (21.781, -13.0119) (21.8009, -13.0238) (21.8411, -13.0468) (21.9025, -13.0791) (21.9865, -13.1178) (22.0943, -13.1605) (22.2042, -13.199) (22.3152, -13.2351) (22.427, -13.2699) (22.5392, -13.3036) (22.652, -13.3363) (22.7653, -13.3676) (22.8795, -13.3969) (22.9947, -13.4241) (23.1107, -13.4492) (23.2275, -13.4723) (23.345, -13.4938) (23.463, -13.5139) (23.5815, -13.5328) (23.7004, -13.5504) (23.8197, -13.5668) (23.9395, -13.5819) (24.0598, -13.5957) (24.1805, -13.608) (24.3017, -13.619) (24.4233, -13.6286) (24.5454, -13.637) (24.6677, -13.6442) (24.7904, -13.6502) (24.9135, -13.6551) (25.0368, -13.6588) (25.1605, -13.6614) (25.2845, -13.6628) (25.4088, -13.663) (25.5334, -13.6621) (25.6582, -13.6601) (25.7833, -13.6569) (25.9087, -13.6527) (26.0342, -13.6474) (26.16, -13.641) (26.2861, -13.6335) (26.4123, -13.625) (26.5388, -13.6154) (26.6654, -13.6048) (26.7922, -13.5932) (26.9192, -13.5805) (27.0464, -13.5668) (27.1737, -13.552) (27.3012, -13.5363) (27.4288, -13.5195) (27.5565, -13.5018) (27.6844, -13.483) (27.8124, -13.4633) (27.9405, -13.4426) (28.0687, -13.4209) (28.1971, -13.3982) (28.3255, -13.3746) (28.454, -13.35) (28.5825, -13.3244) (28.7112, -13.2979) (28.8399, -13.2705) (28.9687, -13.2421) (29.0975, -13.2127) (29.2264, -13.1825) (29.3554, -13.1513) (29.4843, -13.1191) (29.6133, -13.0861) (29.7423, -13.0521) (29.8714, -13.0172) (30.0004, -12.9814) (30.1295, -12.9447) (30.2327, -12.9146) (30.3101, -12.8917) (30.3618, -12.8762) (30.3876, -12.8684) knots 0 0 0 0 0 0 0.01428571 0.02857143 0.04285714 0.05714286 0.07142857 0.08571429 0.1 0.11428571 0.12857143 0.14285714 0.15714286 0.17142857 0.18571429 0.2 0.21428571 0.22857143 0.24285714 0.25714286 0.27142857 0.28571429 0.3 0.31428571 0.32857143 0.34285714 0.35714286 0.37142857 0.38571429 0.4 0.41428571 0.42857143 0.44285714 0.45714286 0.47142857 0.48571429 0.5 0.51428571 0.52857143 0.54285714 0.55714286 0.57142857 0.58571429 0.6 0.61428571 0.62857143 0.64285714 0.65714286 0.67142857 0.68571429 0.7 0.71428571 0.72857143 0.74285714 0.75714286 0.77142857 0.78571429 0.8 0.81428571 0.82857143 0.84285714 0.85714286 0.87142857 0.88571429 0.9 0.91428571 0.92857143 0.94285714 0.95714286 0.97142857 0.98571429 1 1 1 1 1 1
  arc A18 (30.3876, -12.8684) -> (31.5499, -9.675) centre (0, 0) ccw
  spline S9 degree 5 poles (31.5499, -9.675) (31.5351, -9.6525) (31.5055, -9.6074) (31.461, -9.54) (31.4012, -9.4506) (31.3259, -9.3395) (31.2501, -9.2292) (31.1737, -9.1195) (31.0967, -9.0106) (31.0191, -8.9023) (30.941, -8.7948) (30.8623, -8.688) (30.783, -8.582) (30.7032, -8.4767) (30.6228, -8.3722) (30.5418, -8.2684) (30.4603, -8.1654) (30.3782, -8.0632) (30.2956, -7.9617) (30.2124, -7.8611) (30.1287, -7.7612) (30.0444, -7.6622) (29.9596, -7.564) (29.8742, -7.4666) (29.7883, -7.37) (29.7018, -7.2743) (29.6148, -7.1795) (29.5273, -7.0855) (29.4393, -6.9923) (29.3507, -6.9001) (29.2615, -6.8087) (29.1719, -6.7183) (29.0817, -6.6287) (28.991, -6.5401) (28.8998, -6.4525) (28.808, -6.3658) (28.7157, -6.28) (28.623, -6.1952) (28.5297, -6.1114) (28.4358, -6.0286) (28.3415, -5.9467) (28.2467, -5.866) (28.1513, -5.7863) (28.0554, -5.7076) (27.9591, -5.6301) (27.8622, -5.5537) (27.7648, -5.4783) (27.6669, -5.404) (27.5685, -5.3309) (27.4697, -5.2589) (27.3703, -5.1881) (27.2704, -5.1186) (27.17, -5.0504) (27.069, -4.9836) (26.9676, -4.9182) (26.8656, -4.8541) (26.7632, -4.7912) (26.6603, -4.7295) (26.557, -4.669) (26.4531, -4.61) (26.3488, -4.5526) (26.2438, -4.4972) (26.1381, -4.444) (26.0318, -4.3931) (25.9248, -4.3442) (25.8175, -4.2968) (25.7098, -4.2505) (25.6018, -4.2053) (25.4935, -4.1615) (25.3846, -4.1204) (25.2746, -4.0838) (25.1854, -4.0595) (25.1176, -4.0448) (25.072, -4.0366) (25.0491, -4.0329) knots -1 -1 -1 -1 -1 -1 -0.98571429 -0.97142857 -0.95714286 -0.94285714 -0.92857143 -0.91428571 -0.9 -0.88571429 -0.87142857 -0.85714286 -0.84285714 -0.82857143 -0.81428571 -0.8 -0.78571429 -0.77142857 -0.75714286 -0.74285714 -0.72857143 -0.71428571 -0.7 -0.68571429 -0.67142857 -0.65714286 -0.64285714 -0.62857143 -0.61428571 -0.6 -0.58571429 -0.57142857 -0.55714286 -0.54285714 -0.52857143 -0.51428571 -0.5 -0.48571429 -0.47142857 -0.45714286 -0.44285714 -0.42857143 -0.41428571 -0.4 -0.38571429 -0.37142857 -0.35714286 -0.34285714 -0.32857143 -0.31428571 -0.3 -0.28571429 -0.27142857 -0.25714286 -0.24285714 -0.22857143 -0.21428571 -0.2 -0.18571429 -0.17142857 -0.15714286 -0.14285714 -0.12857143 -0.11428571 -0.1 -0.08571429 -0.07142857 -0.05714286 -0.04285714 -0.02857143 -0.01428571 0 0 0 0 0 0
  line L9 (25.0491, -4.0329) -> (21.0066, -3.3807)
  arc A19 (19.6777, -1.6785) -> (21.0066, -3.3807) centre (21.2595, -1.8134) ccw
  arc A20 (19.6777, -1.6785) -> (19.6777, 1.6785) centre (0, 0) ccw
  arc A21 (21.0066, 3.3807) -> (19.6777, 1.6785) centre (21.2595, 1.8134) ccw
  line L10 (21.0066, 3.3807) -> (25.0491, 4.0329)
  spline S10 degree 5 poles (25.0491, 4.0329) (25.072, 4.0366) (25.1176, 4.0448) (25.1854, 4.0595) (25.2746, 4.0838) (25.3846, 4.1204) (25.4935, 4.1615) (25.6018, 4.2053) (25.7098, 4.2505) (25.8175, 4.2968) (25.9248, 4.3442) (26.0318, 4.3931) (26.1381, 4.444) (26.2438, 4.4972) (26.3488, 4.5526) (26.4531, 4.61) (26.557, 4.669) (26.6603, 4.7295) (26.7632, 4.7912) (26.8656, 4.8541) (26.9676, 4.9182) (27.069, 4.9836) (27.17, 5.0504) (27.2704, 5.1186) (27.3703, 5.1881) (27.4697, 5.2589) (27.5685, 5.3309) (27.6669, 5.404) (27.7648, 5.4783) (27.8622, 5.5537) (27.9591, 5.6301) (28.0554, 5.7076) (28.1513, 5.7863) (28.2467, 5.866) (28.3415, 5.9467) (28.4358, 6.0286) (28.5297, 6.1114) (28.623, 6.1952) (28.7157, 6.28) (28.808, 6.3658) (28.8998, 6.4525) (28.991, 6.5401) (29.0817, 6.6287) (29.1719, 6.7183) (29.2615, 6.8087) (29.3507, 6.9001) (29.4393, 6.9923) (29.5273, 7.0855) (29.6148, 7.1795) (29.7018, 7.2743) (29.7883, 7.37) (29.8742, 7.4666) (29.9596, 7.564) (30.0444, 7.6622) (30.1287, 7.7612) (30.2124, 7.8611) (30.2956, 7.9617) (30.3782, 8.0632) (30.4603, 8.1654) (30.5418, 8.2684) (30.6228, 8.3722) (30.7032, 8.4767) (30.783, 8.582) (30.8623, 8.688) (30.941, 8.7948) (31.0191, 8.9023) (31.0967, 9.0106) (31.1737, 9.1195) (31.2501, 9.2292) (31.3259, 9.3395) (31.4012, 9.4506) (31.461, 9.54) (31.5055, 9.6074) (31.5351, 9.6525) (31.5499, 9.675) knots 0 0 0 0 0 0 0.01428571 0.02857143 0.04285714 0.05714286 0.07142857 0.08571429 0.1 0.11428571 0.12857143 0.14285714 0.15714286 0.17142857 0.18571429 0.2 0.21428571 0.22857143 0.24285714 0.25714286 0.27142857 0.28571429 0.3 0.31428571 0.32857143 0.34285714 0.35714286 0.37142857 0.38571429 0.4 0.41428571 0.42857143 0.44285714 0.45714286 0.47142857 0.48571429 0.5 0.51428571 0.52857143 0.54285714 0.55714286 0.57142857 0.58571429 0.6 0.61428571 0.62857143 0.64285714 0.65714286 0.67142857 0.68571429 0.7 0.71428571 0.72857143 0.74285714 0.75714286 0.77142857 0.78571429 0.8 0.81428571 0.82857143 0.84285714 0.85714286 0.87142857 0.88571429 0.9 0.91428571 0.92857143 0.94285714 0.95714286 0.97142857 0.98571429 1 1 1 1 1 1
  arc A22 (31.5499, 9.675) -> (30.3876, 12.8684) centre (0, 0) ccw
  spline S11 degree 5 poles (30.3876, 12.8684) (30.3618, 12.8762) (30.3101, 12.8917) (30.2327, 12.9146) (30.1295, 12.9447) (30.0004, 12.9814) (29.8714, 13.0172) (29.7423, 13.0521) (29.6133, 13.0861) (29.4843, 13.1191) (29.3554, 13.1513) (29.2264, 13.1825) (29.0975, 13.2127) (28.9687, 13.2421) (28.8399, 13.2705) (28.7112, 13.2979) (28.5825, 13.3244) (28.454, 13.35) (28.3255, 13.3746) (28.1971, 13.3982) (28.0687, 13.4209) (27.9405, 13.4426) (27.8124, 13.4633) (27.6844, 13.483) (27.5565, 13.5018) (27.4288, 13.5195) (27.3012, 13.5363) (27.1737, 13.552) (27.0464, 13.5668) (26.9192, 13.5805) (26.7922, 13.5932) (26.6654, 13.6048) (26.5388, 13.6154) (26.4123, 13.625) (26.2861, 13.6335) (26.16, 13.641) (26.0342, 13.6474) (25.9087, 13.6527) (25.7833, 13.6569) (25.6582, 13.6601) (25.5334, 13.6621) (25.4088, 13.663) (25.2845, 13.6628) (25.1605, 13.6614) (25.0368, 13.6588) (24.9135, 13.6551) (24.7904, 13.6502) (24.6677, 13.6442) (24.5454, 13.637) (24.4233, 13.6286) (24.3017, 13.619) (24.1805, 13.608) (24.0598, 13.5957) (23.9395, 13.5819) (23.8197, 13.5668) (23.7004, 13.5504) (23.5815, 13.5328) (23.463, 13.5139) (23.345, 13.4938) (23.2275, 13.4723) (23.1107, 13.4492) (22.9947, 13.4241) (22.8795, 13.3969) (22.7653, 13.3676) (22.652, 13.3363) (22.5392, 13.3036) (22.427, 13.2699) (22.3152, 13.2351) (22.2042, 13.199) (22.0943, 13.1605) (21.9865, 13.1178) (21.9025, 13.0791) (21.8411, 13.0468) (21.8009, 13.0238) (21.781, 13.0119) knots -1 -1 -1 -1 -1 -1 -0.98571429 -0.97142857 -0.95714286 -0.94285714 -0.92857143 -0.91428571 -0.9 -0.88571429 -0.87142857 -0.85714286 -0.84285714 -0.82857143 -0.81428571 -0.8 -0.78571429 -0.77142857 -0.75714286 -0.74285714 -0.72857143 -0.71428571 -0.7 -0.68571429 -0.67142857 -0.65714286 -0.64285714 -0.62857143 -0.61428571 -0.6 -0.58571429 -0.57142857 -0.55714286 -0.54285714 -0.52857143 -0.51428571 -0.5 -0.48571429 -0.47142857 -0.45714286 -0.44285714 -0.42857143 -0.41428571 -0.4 -0.38571429 -0.37142857 -0.35714286 -0.34285714 -0.32857143 -0.31428571 -0.3 -0.28571429 -0.27142857 -0.25714286 -0.24285714 -0.22857143 -0.21428571 -0.2 -0.18571429 -0.17142857 -0.15714286 -0.14285714 -0.12857143 -0.11428571 -0.1 -0.08571429 -0.07142857 -0.05714286 -0.04285714 -0.02857143 -0.01428571 0 0 0 0 0 0
  line L11 (21.781, 13.0119) -> (18.2651, 10.9131)
  arc A23 (16.153, 11.3628) -> (18.2651, 10.9131) centre (17.4514, 12.2762) ccw
  arc A24 (16.153, 11.3628) -> (13.9951, 13.9344) centre (0, 0) ccw
  arc A25 (13.919, 16.0926) -> (13.9951, 13.9344) centre (15.1201, 15.0545) ccw
  line L12 (13.919, 16.0926) -> (16.5965, 19.1906)
  spline S12 degree 5 poles (16.5965, 19.1906) (16.6116, 19.2082) (16.6413, 19.2438) (16.6837, 19.2986) (16.7365, 19.3746) (16.7972, 19.4733) (16.8542, 19.5748) (16.909, 19.678) (16.9627, 19.782) (17.0154, 19.8867) (17.0672, 19.992) (17.1177, 20.0982) (17.1664, 20.2056) (17.2131, 20.3142) (17.258, 20.4242) (17.3011, 20.5352) (17.3426, 20.6472) (17.3829, 20.7599) (17.4221, 20.8733) (17.4601, 20.9873) (17.497, 21.102) (17.5327, 21.2173) (17.5671, 21.3334) (17.6002, 21.4501) (17.632, 21.5676) (17.6626, 21.6857) (17.6921, 21.8044) (17.7204, 21.9237) (17.7477, 22.0435) (17.7738, 22.1638) (17.7989, 22.2847) (17.8229, 22.406) (17.8458, 22.5279) (17.8676, 22.6502) (17.8884, 22.773) (17.908, 22.8963) (17.9267, 23.0201) (17.9443, 23.1443) (17.9608, 23.2689) (17.9764, 23.3939) (17.9909, 23.5193) (18.0045, 23.6451) (18.017, 23.7713) (18.0285, 23.8978) (18.0391, 24.0247) (18.0486, 24.152) (18.0572, 24.2796) (18.0648, 24.4076) (18.0714, 24.5358) (18.0771, 24.6644) (18.0818, 24.7933) (18.0855, 24.9225) (18.0883, 25.052) (18.0902, 25.1818) (18.0911, 25.3118) (18.091, 25.4421) (18.0901, 25.5727) (18.0882, 25.7035) (18.0853, 25.8346) (18.0816, 25.9659) (18.0769, 26.0974) (18.0713, 26.2291) (18.0647, 26.3611) (18.0573, 26.4933) (18.049, 26.6257) (18.0397, 26.7583) (18.0296, 26.8911) (18.0185, 27.024) (18.0066, 27.1571) (17.9937, 27.2904) (17.98, 27.4239) (17.9683, 27.5308) (17.9591, 27.611) (17.9528, 27.6646) (17.9496, 27.6914) knots 0 0 0 0 0 0 0.01428571 0.02857143 0.04285714 0.05714286 0.07142857 0.08571429 0.1 0.11428571 0.12857143 0.14285714 0.15714286 0.17142857 0.18571429 0.2 0.21428571 0.22857143 0.24285714 0.25714286 0.27142857 0.28571429 0.3 0.31428571 0.32857143 0.34285714 0.35714286 0.37142857 0.38571429 0.4 0.41428571 0.42857143 0.44285714 0.45714286 0.47142857 0.48571429 0.5 0.51428571 0.52857143 0.54285714 0.55714286 0.57142857 0.58571429 0.6 0.61428571 0.62857143 0.64285714 0.65714286 0.67142857 0.68571429 0.7 0.71428571 0.72857143 0.74285714 0.75714286 0.77142857 0.78571429 0.8 0.81428571 0.82857143 0.84285714 0.85714286 0.87142857 0.88571429 0.9 0.91428571 0.92857143 0.94285714 0.95714286 0.97142857 0.98571429 1 1 1 1 1 1
  arc A26 (17.9496, 27.6914) -> (15.0066, 29.3905) centre (0, 0) ccw
  spline S13 degree 5 poles (15.0066, 29.3905) (14.9818, 29.3799) (14.9323, 29.3586) (14.8582, 29.3264) (14.7598, 29.2831) (14.6373, 29.2282) (14.5155, 29.1727) (14.3942, 29.1165) (14.2736, 29.0596) (14.1535, 29.002) (14.034, 28.9437) (13.9152, 28.8847) (13.797, 28.8251) (13.6795, 28.7647) (13.5626, 28.7037) (13.4463, 28.642) (13.3307, 28.5796) (13.2158, 28.5165) (13.1016, 28.4528) (12.988, 28.3883) (12.8751, 28.3232) (12.763, 28.2574) (12.6515, 28.1909) (12.5408, 28.1238) (12.4307, 28.0559) (12.3215, 27.9874) (12.2129, 27.9182) (12.1052, 27.8484) (11.9982, 27.7778) (11.8919, 27.7066) (11.7865, 27.6347) (11.6819, 27.5621) (11.578, 27.4888) (11.475, 27.4149) (11.3728, 27.3403) (11.2715, 27.265) (11.171, 27.189) (11.0714, 27.1123) (10.9727, 27.035) (10.8748, 26.957) (10.7779, 26.8783) (10.6818, 26.7989) (10.5868, 26.7189) (10.4927, 26.6381) (10.3996, 26.5566) (10.3075, 26.4745) (10.2164, 26.3917) (10.1262, 26.3082) (10.0371, 26.224) (9.949, 26.1391) (9.8621, 26.0536) (9.7763, 25.9673) (9.6917, 25.8802) (9.6084, 25.7924) (9.5264, 25.7038) (9.4455, 25.6145) (9.3658, 25.5246) (9.2871, 25.434) (9.2097, 25.3427) (9.1335, 25.2507) (9.0589, 25.1579) (8.9861, 25.0641) (8.9154, 24.9693) (8.8467, 24.8734) (8.78, 24.7766) (8.7147, 24.6791) (8.6504, 24.5811) (8.5871, 24.4827) (8.5252, 24.3836) (8.4658, 24.2835) (8.4106, 24.1815) (8.3712, 24.0978) (8.3449, 24.0336) (8.3289, 23.9902) (8.3213, 23.9683) knots -1 -1 -1 -1 -1 -1 -0.98571429 -0.97142857 -0.95714286 -0.94285714 -0.92857143 -0.91428571 -0.9 -0.88571429 -0.87142857 -0.85714286 -0.84285714 -0.82857143 -0.81428571 -0.8 -0.78571429 -0.77142857 -0.75714286 -0.74285714 -0.72857143 -0.71428571 -0.7 -0.68571429 -0.67142857 -0.65714286 -0.64285714 -0.62857143 -0.61428571 -0.6 -0.58571429 -0.57142857 -0.55714286 -0.54285714 -0.52857143 -0.51428571 -0.5 -0.48571429 -0.47142857 -0.45714286 -0.44285714 -0.42857143 -0.41428571 -0.4 -0.38571429 -0.37142857 -0.35714286 -0.34285714 -0.32857143 -0.31428571 -0.3 -0.28571429 -0.27142857 -0.25714286 -0.24285714 -0.22857143 -0.21428571 -0.2 -0.18571429 -0.17142857 -0.15714286 -0.14285714 -0.12857143 -0.11428571 -0.1 -0.08571429 -0.07142857 -0.05714286 -0.04285714 -0.02857143 -0.01428571 0 0 0 0 0 0
  line L13 (8.3213, 23.9683) -> (6.9771, 20.1005)
  arc A27 (5.07, 19.0873) -> (6.9771, 20.1005) centre (5.4776, 20.6216) ccw
  arc A28 (5.07, 19.0873) -> (1.764, 19.6703) centre (0, 0) ccw
  arc A29 (0.3185, 21.2746) -> (1.764, 19.6703) centre (1.9058, 21.2514) ccw
  line L14 (0.3185, 21.2746) -> (0.3781, 25.3689)
  spline S14 degree 5 poles (0.3781, 25.3689) (0.3785, 25.3921) (0.3783, 25.4384) (0.3756, 25.5077) (0.3671, 25.5998) (0.3502, 25.7145) (0.3286, 25.8289) (0.3043, 25.9431) (0.2785, 26.0573) (0.2517, 26.1714) (0.2236, 26.2853) (0.194, 26.3991) (0.1623, 26.5127) (0.1283, 26.626) (0.092, 26.739) (0.0536, 26.8518) (0.0135, 26.9643) (-0.0281, 27.0765) (-0.071, 27.1885) (-0.1152, 27.3003) (-0.1606, 27.4119) (-0.2074, 27.5232) (-0.2557, 27.6342) (-0.3054, 27.7449) (-0.3565, 27.8554) (-0.4089, 27.9655) (-0.4627, 28.0754) (-0.5176, 28.185) (-0.5738, 28.2943) (-0.6311, 28.4033) (-0.6895, 28.512) (-0.7492, 28.6203) (-0.8099, 28.7284) (-0.8719, 28.8362) (-0.935, 28.9436) (-0.9991, 29.0507) (-1.0644, 29.1575) (-1.1308, 29.2639) (-1.1981, 29.37) (-1.2666, 29.4758) (-1.3361, 29.5812) (-1.4065, 29.6862) (-1.4781, 29.791) (-1.5506, 29.8953) (-1.6241, 29.9993) (-1.6986, 30.1029) (-1.774, 30.2062) (-1.8504, 30.3091) (-1.9278, 30.4116) (-2.0061, 30.5138) (-2.0854, 30.6155) (-2.1656, 30.7169) (-2.2466, 30.8179) (-2.3286, 30.9185) (-2.4115, 31.0187) (-2.4953, 31.1185) (-2.58, 31.2179) (-2.6656, 31.3169) (-2.752, 31.4154) (-2.8393, 31.5136) (-2.9274, 31.6113) (-3.0164, 31.7087) (-3.1062, 31.8056) (-3.1969, 31.9021) (-3.2884, 31.9981) (-3.3807, 32.0937) (-3.4738, 32.1889) (-3.5677, 32.2837) (-3.6624, 32.378) (-3.758, 32.4718) (-3.8543, 32.5652) (-3.932, 32.6396) (-3.9906, 32.6952) (-4.0298, 32.7321) (-4.0495, 32.7506) knots 0 0 0 0 0 0 0.01428571 0.02857143 0.04285714 0.05714286 0.07142857 0.08571429 0.1 0.11428571 0.12857143 0.14285714 0.15714286 0.17142857 0.18571429 0.2 0.21428571 0.22857143 0.24285714 0.25714286 0.27142857 0.28571429 0.3 0.31428571 0.32857143 0.34285714 0.35714286 0.37142857 0.38571429 0.4 0.41428571 0.42857143 0.44285714 0.45714286 0.47142857 0.48571429 0.5 0.51428571 0.52857143 0.54285714 0.55714286 0.57142857 0.58571429 0.6 0.61428571 0.62857143 0.64285714 0.65714286 0.67142857 0.68571429 0.7 0.71428571 0.72857143 0.74285714 0.75714286 0.77142857 0.78571429 0.8 0.81428571 0.82857143 0.84285714 0.85714286 0.87142857 0.88571429 0.9 0.91428571 0.92857143 0.94285714 0.95714286 0.97142857 0.98571429 1 1 1 1 1 1
  arc A30 (-4.0495, 32.7506) -> (-7.3961, 32.1605) centre (0, 0) ccw
  spline S15 degree 5 poles (-7.3961, 32.1605) (-7.4083, 32.1364) (-7.4325, 32.0883) (-7.4686, 32.016) (-7.5161, 31.9195) (-7.5747, 31.7988) (-7.6323, 31.678) (-7.6891, 31.557) (-7.745, 31.4358) (-7.7999, 31.3145) (-7.854, 31.1931) (-7.9071, 31.0715) (-7.9593, 30.9499) (-8.0105, 30.8281) (-8.0609, 30.7062) (-8.1103, 30.5842) (-8.1587, 30.4621) (-8.2062, 30.3399) (-8.2527, 30.2176) (-8.2983, 30.0953) (-8.3429, 29.9728) (-8.3865, 29.8503) (-8.4292, 29.7277) (-8.4708, 29.6051) (-8.5115, 29.4824) (-8.5512, 29.3597) (-8.5898, 29.2369) (-8.6275, 29.1141) (-8.6641, 28.9913) (-8.6997, 28.8685) (-8.7342, 28.7456) (-8.7677, 28.6227) (-8.8002, 28.4999) (-8.8316, 28.377) (-8.8619, 28.2542) (-8.8911, 28.1313) (-8.9192, 28.0086) (-8.9463, 27.8858) (-8.9722, 27.7631) (-8.997, 27.6404) (-9.0207, 27.5178) (-9.0432, 27.3953) (-9.0646, 27.2729) (-9.0848, 27.1506) (-9.1037, 27.0283) (-9.1215, 26.9062) (-9.138, 26.7842) (-9.1534, 26.6623) (-9.1676, 26.5405) (-9.1805, 26.4189) (-9.1921, 26.2974) (-9.2024, 26.1762) (-9.2112, 26.0551) (-9.2186, 25.9343) (-9.2245, 25.8137) (-9.229, 25.6933) (-9.2323, 25.5732) (-9.2343, 25.4532) (-9.235, 25.3335) (-9.2342, 25.2141) (-9.2317, 25.095) (-9.2272, 24.9764) (-9.2204, 24.8583) (-9.2113, 24.7407) (-9.2003, 24.6237) (-9.1876, 24.507) (-9.1738, 24.3906) (-9.159, 24.2745) (-9.1428, 24.1588) (-9.1239, 24.0439) (-9.1006, 23.9303) (-9.0771, 23.8409) (-9.0559, 23.7749) (-9.0402, 23.7313) (-9.032, 23.7096) knots -1 -1 -1 -1 -1 -1 -0.98571429 -0.97142857 -0.95714286 -0.94285714 -0.92857143 -0.91428571 -0.9 -0.88571429 -0.87142857 -0.85714286 -0.84285714 -0.82857143 -0.81428571 -0.8 -0.78571429 -0.77142857 -0.75714286 -0.74285714 -0.72857143 -0.71428571 -0.7 -0.68571429 -0.67142857 -0.65714286 -0.64285714 -0.62857143 -0.61428571 -0.6 -0.58571429 -0.57142857 -0.55714286 -0.54285714 -0.52857143 -0.51428571 -0.5 -0.48571429 -0.47142857 -0.45714286 -0.44285714 -0.42857143 -0.41428571 -0.4 -0.38571429 -0.37142857 -0.35714286 -0.34285714 -0.32857143 -0.31428571 -0.3 -0.28571429 -0.27142857 -0.25714286 -0.24285714 -0.22857143 -0.21428571 -0.2 -0.18571429 -0.17142857 -0.15714286 -0.14285714 -0.12857143 -0.11428571 -0.1 -0.08571429 -0.07142857 -0.05714286 -0.04285714 -0.02857143 -0.01428571 0 0 0 0 0 0
  line L15 (-9.032, 23.7096) -> (-7.5756, 19.8826)
  arc A31 (-8.3852, 17.8807) -> (-7.5756, 19.8826) centre (-9.0593, 19.318) ccw
  arc A32 (-8.3852, 17.8807) -> (-11.2925, 16.2022) centre (0, 0) ccw
  arc A33 (-13.4311, 16.502) -> (-11.2925, 16.2022) centre (-12.2002, 17.5045) ccw
  line L16 (-13.4311, 16.502) -> (-16.0171, 19.6768)
  spline S16 degree 5 poles (-16.0171, 19.6768) (-16.0318, 19.6947) (-16.0617, 19.7301) (-16.1083, 19.7814) (-16.174, 19.8466) (-16.2607, 19.9235) (-16.3507, 19.9973) (-16.4428, 20.0692) (-16.5359, 20.1401) (-16.6299, 20.2102) (-16.7246, 20.2795) (-16.8204, 20.3476) (-16.9177, 20.4142) (-17.0166, 20.4792) (-17.1171, 20.5424) (-17.2189, 20.6041) (-17.322, 20.6645) (-17.426, 20.7237) (-17.5309, 20.782) (-17.6365, 20.8392) (-17.7431, 20.8955) (-17.8505, 20.9506) (-17.9588, 21.0047) (-18.068, 21.0576) (-18.1782, 21.1093) (-18.2892, 21.16) (-18.401, 21.2096) (-18.5135, 21.2582) (-18.6267, 21.3059) (-18.7407, 21.3525) (-18.8553, 21.3982) (-18.9707, 21.4429) (-19.0867, 21.4866) (-19.2034, 21.5293) (-19.3208, 21.5711) (-19.4388, 21.6119) (-19.5574, 21.6517) (-19.6767, 21.6906) (-19.7965, 21.7286) (-19.9169, 21.7656) (-20.0379, 21.8017) (-20.1594, 21.8369) (-20.2815, 21.8711) (-20.4041, 21.9045) (-20.5273, 21.9369) (-20.651, 21.9684) (-20.7752, 21.999) (-20.8998, 22.0287) (-21.025, 22.0575) (-21.1507, 22.0854) (-21.2768, 22.1124) (-21.4034, 22.1385) (-21.5304, 22.1638) (-21.6579, 22.1881) (-21.7858, 22.2116) (-21.9141, 22.2342) (-22.0429, 22.2559) (-22.172, 22.2767) (-22.3016, 22.2967) (-22.4315, 22.3158) (-22.5619, 22.334) (-22.6926, 22.3514) (-22.8237, 22.3679) (-22.9552, 22.3835) (-23.087, 22.3983) (-23.2192, 22.4122) (-23.3517, 22.4252) (-23.4846, 22.4374) (-23.6177, 22.4488) (-23.7512, 22.4593) (-23.8851, 22.4689) (-23.9924, 22.476) (-24.073, 22.4809) (-24.1268, 22.484) (-24.1537, 22.4855) knots 0 0 0 0 0 0 0.01428571 0.02857143 0.04285714 0.05714286 0.07142857 0.08571429 0.1 0.11428571 0.12857143 0.14285714 0.15714286 0.17142857 0.18571429 0.2 0.21428571 0.22857143 0.24285714 0.25714286 0.27142857 0.28571429 0.3 0.31428571 0.32857143 0.34285714 0.35714286 0.37142857 0.38571429 0.4 0.41428571 0.42857143 0.44285714 0.45714286 0.47142857 0.48571429 0.5 0.51428571 0.52857143 0.54285714 0.55714286 0.57142857 0.58571429 0.6 0.61428571 0.62857143 0.64285714 0.65714286 0.67142857 0.68571429 0.7 0.71428571 0.72857143 0.74285714 0.75714286 0.77142857 0.78571429 0.8 0.81428571 0.82857143 0.84285714 0.85714286 0.87142857 0.88571429 0.9 0.91428571 0.92857143 0.94285714 0.95714286 0.97142857 0.98571429 1 1 1 1 1 1
  arc A34 (-24.1537, 22.4855) -> (-26.3381, 19.8822) centre (0, 0) ccw